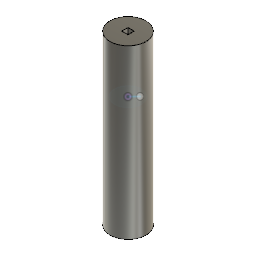
motor shaft to bridge connector (Autodesk Fusion 360 design; units mm, degrees)
Autodesk Fusion 360 part; units mm, degrees
sketch "Sketch1" plane through (0, 0, 0) normal (0, 0, 1) x (1, 0, 0)
sketch "Sketch2" plane through (0, 0, 0) normal (0, 0, 1) x (1, 0, 0)
  circle A0 centre (0, 0) radius 3.5
  dimension "d1" = 7
  constraint coincident A0.centre origin
  measures "d1" diameter of A0
extrude "Extrude6" add sketch "Sketch2" along normal blind 32.5
sketch "Sketch7" plane through (0, 0, 0) normal (0, 0, 1) x (1, 0, 0)
  circle A0 centre (0, 0) radius 2.6
  dimension "d22" = 5.2
  constraint coincident A0.centre origin
  measures "d22" diameter of A0
extrude "Extrude7" cut sketch "Sketch7" along normal blind 21.5
sketch "Sketch8" plane through (0, 0, 0) normal (0, 1, 0) x (1, 0, 0)
  line L0 (0, 0) -> (0, -10)
  circle A0 centre (0, -10) radius 1.6
  dimension "d25" = 10
  dimension "d26" = 3.2
  constraint coincident L0.start origin
  constraint vertical L0
  constraint coincident L0.end A0.centre
  measures "d25" distance of L0.start L0.end
  measures "d26" diameter of A0
extrude "Extrude8" cut sketch "Sketch8" against normal blind 3.5
sketch "Sketch9" plane through (0, 0, 0) normal (0, 1, 0) x (1, 0, 0)
  line L0 (0, -32) -> (0, -26)
  circle A0 centre (0, -26) radius 1.6
  dimension "d29" = 6
  dimension "d30" = 3.2
  constraint vertical L0
  constraint coincident L0.end A0.centre
  measures "d29" distance of L0.start L0.end
  measures "d30" diameter of A0
extrude "Extrude9" cut sketch "Sketch9" against normal blind 3.5
sketch "Sketch10" plane through (0, 0, 21.5) normal (0, 0, -1) x (1, 0, 0)
  circle A0 centre (0, 0) radius 2.6
  line L0 (0, 0) -> (1.126, -1.2061)
  dimension "d33" = 1.65
  constraint coincident A0.centre L0.start
  measures "d33" distance of A0.centre L0.end
sketch "Sketch18" plane through (0, 0, 32.5) normal (0, 0, 1) x (-1, 0, 0)
  circle A0 centre (0, 0) radius 3.5
  line L0 (0.6, -0.6) -> (-0.6, -0.6)
  line L1 (-0.6, -0.6) -> (-0.6, 0.6)
  line L2 (-0.6, 0.6) -> (0.6, 0.6)
  line L3 (0.6, 0.6) -> (0.6, -0.6)
  line L4 (0.6, -0.6) -> (-0.6, 0.6) construction
  line L5 (-0.6, -0.6) -> (0.6, 0.6) construction
  dimension "d40" = 1.2
  dimension "d41" = 1.2
  constraint horizontal L0
  constraint perpendicular L0 L1
  constraint parallel L0 L2
  constraint parallel L1 L3
  constraint coincident L4 A0.centre
  constraint coincident L5 A0.centre
  constraint coincident A0.centre origin
  measures "d40" distance of L1.end L2.end
  measures "d41" distance of L0.end L1.end
extrude "Extrude10" cut sketch "Sketch18" against normal blind 15 contours L0 L1 L2 L3
delete_face "DeleteFace1" 1 faces at (-0.7412, -1.3353, 24.582)
delete_face "DeleteFace2" 1 faces at (1.3379, -2.5658, 10.8775)
